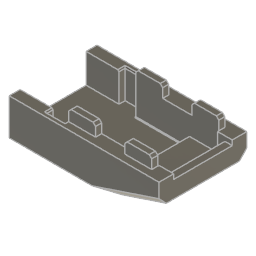
DiabolicParasite-Case-Top (Autodesk Fusion 360 design; units mm, degrees)
Autodesk Fusion 360 part; units mm, degrees
sketch "Skizze1" plane through (0, 0, 0) normal (0, 0, 1) x (1, 0, 0)
  line L0 (0, 0) -> (30.7, 0)
  line L1 (30.7, 0) -> (30.7, 18)
  line L2 (30.7, 18) -> (0, 18)
  line L3 (0, 18) -> (0, 0)
  dimension "d1" = 30.7
  dimension "d2" = 18
  constraint horizontal L0
  constraint vertical L1
  constraint horizontal L2
  constraint vertical L3
  constraint coincident L0.start L3.end
  measures "d1" distance of L0.start L0.end
  measures "d2" distance of L0.start L2.end
extrude "Extrusion1" add sketch "Skizze1" along normal blind 1.5
sketch "Skizze2" plane through (0, 0, 1.5) normal (0, 0, 1) x (-1, 0, 0)
  line L0 (0, -18) -> (0, 0)
  line L1 (0, 0) -> (-30.7, 0)
  line L2 (-30.7, 0) -> (-30.7, -18)
  line L3 (-30.7, -18) -> (0, -18)
  line L4 (-30.7, -18) -> (-10.7, -18)
  line L5 (-10.7, -18) -> (-10.7, -15)
  line L6 (-10.7, -15) -> (-30.7, -15)
  line L7 (-30.7, -15) -> (-30.7, -18)
  line L8 (-30.7, 0) -> (-10.7, 0)
  line L9 (-10.7, 0) -> (-10.7, -3)
  line L10 (-10.7, -3) -> (-30.7, -3)
  line L11 (-30.7, -3) -> (-30.7, 0)
  dimension "d5" = 20
  dimension "d6" = 3
  dimension "d7" = 20
  dimension "d8" = 3
  constraint horizontal L4
  constraint vertical L5
  constraint horizontal L6
  constraint vertical L7
  constraint coincident L2.end L3.start
  constraint horizontal L8
  constraint vertical L9
  constraint horizontal L10
  constraint vertical L11
  constraint coincident L1.end L2.start
  measures "d5" distance of L2.end L4.end
  measures "d6" distance of L2.end L6.end
  measures "d7" distance of L1.end L8.end
  measures "d8" distance of L1.end L10.end
extrude "Extrusion2" add sketch "Skizze2" along normal blind 6 contours L2 L3 L4 L5 L6 L7 | L1 L2 L8 L9 L10 L11
sketch "Skizze3" plane through (0, 0, 1.5) normal (0, 0, 1) x (-1, 0, 0)
  line L0 (-10.7, 0) -> (-10.7, -3)
  line L1 (-10.7, -3) -> (-30.7, -3)
  line L2 (-30.7, -3) -> (-30.7, -15)
  line L3 (-30.7, -15) -> (-10.7, -15)
  line L4 (-10.7, -15) -> (-10.7, -18)
  line L5 (-10.7, -18) -> (0, -18)
  line L6 (0, -18) -> (0, 0)
  line L7 (0, 0) -> (-10.7, 0)
  line L8 (-10.7, -18) -> (-10.7, -17)
  line L9 (-10.7, -17) -> (-7.5, -17)
  line L10 (-7.5, -17) -> (-7.5, -15.25)
  line L11 (-7.5, -15.25) -> (0, -15.25)
  line L12 (0, -15.25) -> (0, -18)
  line L13 (0, -18) -> (-10.7, -18)
  line L14 (-30.7, -9) -> (0.9, -9)
  line L15 (0, 0) -> (-10.7, 0)
  line L16 (0, -2.75) -> (0, 0)
  line L17 (-7.5, -2.75) -> (0, -2.75)
  line L18 (-7.5, -1) -> (-7.5, -2.75)
  line L19 (-10.7, -1) -> (-7.5, -1)
  line L20 (-10.7, 0) -> (-10.7, -1)
  dimension "d11" = 1
  dimension "d12" = 3.2
  dimension "d13" = 1.75
  constraint coincident L4.end L5.start
  constraint perpendicular L3 L8
  constraint perpendicular L4 L9
  constraint perpendicular L9 L10
  constraint coincident L6 L11.end
  constraint perpendicular L6 L11
  constraint coincident L5.end L6.start
  constraint midpoint L2 L14.start
  constraint perpendicular L6 L14
  constraint symmetric L4.end L14 L0.start
  constraint symmetric L8.end L14 L19.start
  constraint symmetric L9.end L14 L18.start
  constraint symmetric L10.end L14 L17.start
  constraint symmetric L11.end L14 L16.start
  constraint symmetric L5.end L14 L6.end
  measures "d11" distance of L4.end L8.end
  measures "d12" distance of L8.end L9.end
  measures "d13" distance of L9.end L10.end L6.end
extrude "Extrusion3" add sketch "Skizze3" along normal blind 6 contours L0 L6 L7 L15 L16 L17 L18 L19 L20 | L4 L5 L6 L8 L9 L10 L11 L12 L13
sketch "Skizze4" plane through (0, 0, 7.5) normal (0, 0, 1) x (-1, 0, 0)
  line L0 (-30.7, -15) -> (-30.7, -18)
  line L1 (-30.7, -18) -> (0, -18)
  line L2 (0, -18) -> (0, -15.25)
  line L3 (0, -15.25) -> (-7.5, -15.25)
  line L4 (-7.5, -15.25) -> (-7.5, -17)
  line L5 (-7.5, -17) -> (-10.7, -17)
  line L6 (-10.7, -17) -> (-10.7, -15)
  line L7 (-10.7, -15) -> (-30.7, -15)
sketch "Skizze5" plane through (0, 0, 7.5) normal (0, 0, 1) x (-1, 0, 0)
  line L0 (-10.7, -15) -> (-27.7, -15)
  line L1 (-27.7, -15) -> (-27.7, -16.5)
  line L2 (-27.7, -16.5) -> (-10.7, -16.5)
  line L3 (-10.7, -16.5) -> (-10.7, -15)
  line L4 (0, -18) -> (0, 0)
  line L5 (-27.7, -1.5) -> (-10.7, -1.5)
  line L6 (-10.7, -1.5) -> (-10.7, -3)
  line L7 (-10.7, -3) -> (-27.7, -3)
  line L8 (-27.7, -3) -> (-27.7, -1.5)
  point P0 (-30.7, -15)
  dimension "d18" = 17
  dimension "d19" = 1.5
  dimension "d20" = 3
  constraint horizontal L0
  constraint vertical L1
  constraint horizontal L2
  constraint vertical L3
  constraint coincident L4.end origin
  constraint perpendicular L0 L4
  measures "d18" distance of L0.start L0.end
  measures "d19" distance of L0.start L2.end
  measures "d20" distance of L0.end P0
extrude "Extrusion4" add sketch "Skizze5" along normal blind 2.4
chamfer "Fase1" distance 0.5 angle 45 4 edges at (10.7, 15.75, 9.9) (27.7, 15.75, 9.9) (10.7, 2.25, 9.9) (27.7, 2.25, 9.9)
extrude "Extrusion5" cut 1 faces at (2.5, 15.25, 5.5) along direction (0, 1, 0) blind 0.25
extrude "Extrusion6" cut 1 faces at (5, 2.75, 3.5) along direction (0, -1, 0) blind 0.25
sketch "Skizze6" plane through (0, 0, 1.5) normal (0, 0, 1) x (-1, 0, 0)
  line L0 (-7.5, -1) -> (-10.7, -1)
  line L1 (-10.7, -1) -> (-10.7, -3)
  line L2 (-10.7, -3) -> (-30.7, -3)
  line L3 (-30.7, -3) -> (-30.7, -15)
  line L4 (-30.7, -15) -> (-10.7, -15)
  line L5 (-10.7, -15) -> (-10.7, -17)
  line L6 (-10.7, -17) -> (-7.5, -17)
  line L7 (-7.5, -17) -> (-7.5, -15.5)
  line L8 (-7.5, -15.5) -> (0, -15.5)
  line L9 (0, -15.5) -> (0, -2.5)
  line L10 (0, -2.5) -> (-7.5, -2.5)
  line L11 (-7.5, -2.5) -> (-7.5, -1)
  line L12 (-30.7, -3) -> (-29.2, -3)
  line L13 (-29.2, -3) -> (-29.2, -15)
  line L14 (-29.2, -15) -> (-30.7, -15)
  line L15 (-30.7, -15) -> (-30.7, -3)
  dimension "d28" = 1.5
  constraint horizontal L12
  constraint vertical L13
  constraint horizontal L14
  constraint vertical L15
  constraint coincident L4 L13.end
  constraint coincident L2.end L3.start
  measures "d28" distance of L2.end L12.end
extrude "Extrusion7" add sketch "Skizze6" along normal blind 5 contours L2 L3 L4 L12 L13 L14 L15
extrude "Extrusion8" cut 1 faces at (7.5, 2, 5.5) along direction (-1, 0, 0) blind 0.5
extrude "Extrusion9" cut 1 faces at (7.5, 16.5, 3.5) along direction (-1, 0, 0) blind 0.5
extrude "Extrusion10" cut 1 faces at (4.6667, 15.5, 5.5) along direction (0, 1, 0) blind 0.25
extrude "Extrusion11" cut 1 faces at (4.6667, 2.5, 5.5) along direction (0, -1, 0) blind 0.25
sketch "Skizze7" plane through (0, 3, 0) normal (0, 1, 0) x (-1, 0, 0)
  line L0 (-30.7, 6.5) -> (-29.2, 6.5)
  line L1 (-29.2, 6.5) -> (-29.2, 1.5)
  line L2 (-29.2, 1.5) -> (-10.7, 1.5)
  line L3 (-10.7, 1.5) -> (-10.7, 9.4)
  line L4 (-10.7, 9.4) -> (-11.2, 9.9)
  line L5 (-11.2, 9.9) -> (-27.2, 9.9)
  line L6 (-27.2, 9.9) -> (-27.7, 9.4)
  line L7 (-27.7, 9.4) -> (-27.7, 7.5)
  line L8 (-27.7, 7.5) -> (-30.7, 7.5)
  line L9 (-30.7, 7.5) -> (-30.7, 6.5)
  line L10 (-27.7, 9.4) -> (-27.2, 9.9)
  line L11 (-27.2, 9.9) -> (-11.2, 9.9)
  line L12 (-11.2, 9.9) -> (-10.7, 9.4)
  line L13 (-10.7, 9.4) -> (-10.7, 1.5)
  line L14 (-27.7, 9.4) -> (-27.7, 1.5)
  line L15 (-27.7, 1.5) -> (-10.7, 1.5)
  constraint coincident L6.end L7.start
  constraint coincident L5.end L6.start
  constraint coincident L4.end L5.start
  constraint coincident L3.end L4.start
  constraint coincident L2.end L3.start
  constraint coincident L2 L14.end
  constraint perpendicular L2 L14
extrude "Extrusion12" cut sketch "Skizze7" against normal blind 0.25 contours L2 L3 L4 L5 L6 L7 L10 L11 L12 L13 L14 L15
sketch "Skizze8" plane through (0, 15, 0) normal (0, -1, 0) x (1, 0, 0)
  line L0 (29.2, 1.5) -> (29.2, 6.5)
  line L1 (29.2, 6.5) -> (30.7, 6.5)
  line L2 (30.7, 6.5) -> (30.7, 7.5)
  line L3 (30.7, 7.5) -> (27.7, 7.5)
  line L4 (27.7, 7.5) -> (27.7, 9.4)
  line L5 (27.7, 9.4) -> (27.2, 9.9)
  line L6 (27.2, 9.9) -> (11.2, 9.9)
  line L7 (11.2, 9.9) -> (10.7, 9.4)
  line L8 (10.7, 9.4) -> (10.7, 1.5)
  line L9 (10.7, 1.5) -> (29.2, 1.5)
  line L10 (27.7, 7.5) -> (27.7, 1.5)
  line L11 (27.7, 1.5) -> (10.7, 1.5)
  line L12 (10.7, 1.5) -> (10.7, 9.4)
  line L13 (10.7, 9.4) -> (11.2, 9.9)
  line L14 (11.2, 9.9) -> (27.2, 9.9)
  line L15 (27.2, 9.9) -> (27.7, 9.4)
  line L16 (27.7, 9.4) -> (27.7, 7.5)
extrude "Extrusion13" cut sketch "Skizze8" against normal blind 0.25 contours L4 L5 L6 L7 L8 L9 L10 L11 L12 L13 L14 L15 L16
extrude "Extrusion14" cut 1 faces at (7, 1.4167, 3.5) along direction (-1, 0, 0) blind 0.25
extrude "Extrusion15" cut 1 faces at (7, 16.5833, 3.5) along direction (-1, 0, 0) blind 0.25
chamfer "Fase3" distance 0.25 angle 45 4 edges at (8.725, 1, 7.5) (6.75, 1.625, 7.5) (6.75, 16.375, 7.5) (8.725, 17, 7.5)
sketch "Skizze9" plane through (0, 0, 9.9) normal (0, 0, 1) x (-1, 0, 0)
  line L0 (-27.2, -2.75) -> (-11.2, -2.75)
  line L1 (-11.2, -2.75) -> (-11.2, -1.5)
  line L2 (-11.2, -1.5) -> (-27.2, -1.5)
  line L3 (-27.2, -1.5) -> (-27.2, -2.75)
  line L4 (-22.2, -2.75) -> (-16.2, -2.75)
  line L5 (-16.2, -2.75) -> (-16.2, -1.5)
  line L6 (-16.2, -1.5) -> (-22.2, -1.5)
  line L7 (-22.2, -1.5) -> (-22.2, -2.75)
  line L8 (-22.2, -16.5) -> (-16.2, -16.5)
  line L9 (-16.2, -16.5) -> (-16.2, -15.25)
  line L10 (-16.2, -15.25) -> (-22.2, -15.25)
  line L11 (-22.2, -15.25) -> (-22.2, -16.5)
  point P0 (-27.7, -2.75)
  dimension "d49" = 6
  dimension "d50" = 5.5
  dimension "d51" = 1.25
  constraint horizontal L4
  constraint vertical L5
  constraint horizontal L6
  constraint vertical L7
  constraint coincident L2 L5.end
  constraint coincident L0 L4.start
  constraint horizontal L8
  constraint vertical L9
  constraint horizontal L10
  constraint vertical L11
  measures "d49" distance of L5 L7
  measures "d50" distance of L4.start P0
  measures "d51" distance of L8.start L10.end
extrude "Extrusion16" cut sketch "Skizze9" against normal blind 2.4 contours L0 L2 L4 L5 L6 L7 | L8 L9 L10 L11
chamfer "Fase4" distance 0.5 angle 45 4 edges at (22.2, 2.125, 9.9) (16.2, 2.125, 9.9) (16.2, 15.875, 9.9) (22.2, 15.875, 9.9)
sketch "Skizze10" plane through (0, 0, 1.5) normal (0, 0, 1) x (-1, 0, 0)
  line L0 (-29.2, -3) -> (-29.2, -15)
  line L1 (-29.2, -15) -> (-27.7, -15)
  line L2 (-27.7, -15) -> (-10.7, -15)
  line L3 (-10.7, -15) -> (-10.7, -15.25)
  line L4 (-10.7, -15.25) -> (-10.7, -17)
  line L5 (-10.7, -17) -> (-6.75, -17)
  line L6 (-6.75, -17) -> (-6.75, -15.75)
  line L7 (-6.75, -15.75) -> (0, -15.75)
  line L8 (0, -15.75) -> (0, -2.25)
  line L9 (0, -2.25) -> (-6.75, -2.25)
  line L10 (-6.75, -2.25) -> (-6.75, -1)
  line L11 (-6.75, -1) -> (-10.7, -1)
  line L12 (-10.7, -1) -> (-10.7, -2.75)
  line L13 (-10.7, -2.75) -> (-10.7, -3)
  line L14 (-10.7, -3) -> (-27.7, -3)
  line L15 (-27.7, -3) -> (-29.2, -3)
  line L16 (-29.2, -3) -> (-27.7, -3)
  line L17 (-27.7, -2.75) -> (-21.7, -2.75)
  line L18 (-29.2, -3) -> (-29.2, -15)
  line L19 (-29.2, -15) -> (-27.7, -15)
  line L20 (-27.7, -15) -> (-27.7, -15.25)
  line L21 (-27.7, -15.25) -> (-21.7, -15.25)
  line L22 (-21.7, -15.25) -> (-21.7, -2.75)
  line L23 (-27.7, -3) -> (-27.7, -2.75)
  dimension "d55" = 6
  dimension "d56" = 6
  constraint coincident L0.start L15.end
  constraint coincident L14.end L15.start
  constraint perpendicular L0 L17
  constraint coincident L0.end L1.start
  constraint coincident L1.end L2.start
  constraint perpendicular L1 L20
  constraint perpendicular L20 L21
  measures "d55" distance of L17.start L17.end
  measures "d56" distance of L20.end L21.end
extrude "Extrusion18" add sketch "Skizze10" along normal blind 2 contours L0 L1 L2 L14 L15 L16 L18 L19 L22 | L14 L17 L22 L23 | L2 L20 L21 L22
chamfer "Fase6" distance 3 distance2 9 1 edges at (30.7, 9, 0) measured on face at (30.7, 7, 2.1667)
chamfer "Fase7" distance 1.5 angle 45 2 edges at (26.2, 0, 1.5) (26.2, 18, 1.5)
sketch "Skizze11" plane through (0, 0, 0) normal (0, 0, -1) x (1, 0, 0)
  line L0 (16.9566, -18) -> (21.7, -16.5)
  line L1 (21.7, -16.5) -> (21.7, -1.5)
  line L2 (21.7, -1.5) -> (16.9566, 0)
  line L3 (16.9566, 0) -> (0, 0)
  line L4 (0, 0) -> (0, -18)
  line L5 (0, -18) -> (16.9566, -18)
  line L6 (1.2141, -8.8075) -> (4.2737, -10.5308)
  line L7 (4.2737, -10.5308) -> (4.2721, -9.2547)
  line L8 (4.2721, -9.2547) -> (13.5116, -9.2746)
  spline S0 degree 3 poles (13.5116, -9.2746) (13.4697, -9.4576) (13.3762, -9.6062) (13.3229, -9.7697) knots 0 0 0 0 1 1 1 1
  spline S1 degree 3 poles (13.3229, -9.7697) (13.022, -10.6918) (12.4198, -11.2426) (11.3356, -11.2485) knots 0 0 0 0 1 1 1 1
  line L9 (11.3356, -11.2485) -> (10.5675, -11.2692)
  spline S2 degree 3 poles (10.5675, -11.2692) (10.4017, -11.0954) (10.4168, -10.9819) (10.3217, -10.8317) knots 0 0 0 0 1 1 1 1
  spline S3 degree 3 poles (10.3217, -10.8317) (10.1903, -10.6244) (9.9419, -10.4277) (9.7381, -10.3457) knots 0 0 0 0 1 1 1 1
  spline S4 degree 3 poles (9.7381, -10.3457) (8.6591, -9.911) (7.5802, -10.5592) (7.5399, -11.7608) knots 0 0 0 0 1 1 1 1
  spline S5 degree 3 poles (7.5399, -11.7608) (7.6724, -13.4837) (9.8775, -13.9287) (10.5675, -12.1456) knots 0 0 0 0 1 1 1 1
  line L10 (10.5675, -12.1456) -> (11.6596, -12.1144)
  spline S6 degree 3 poles (11.6596, -12.1144) (12.302, -12.0867) (12.8976, -11.8491) (13.4441, -11.3899) knots 0 0 0 0 1 1 1 1
  spline S7 degree 3 poles (13.4441, -11.3899) (13.7999, -10.8974) (14.1556, -10.1496) (14.5114, -9.2735) knots 0 0 0 0 1 1 1 1
  line L11 (14.5114, -9.2735) -> (16.956, -9.2513)
  spline S8 degree 3 poles (16.956, -9.2513) (17.2824, -10.0163) (17.8277, -10.2894) (18.4423, -10.2766) knots 0 0 0 0 1 1 1 1
  spline S9 degree 3 poles (18.4423, -10.2766) (19.2203, -10.2605) (20.0125, -9.5959) (19.9455, -8.7505) knots 0 0 0 0 1 1 1 1
  spline S10 degree 3 poles (19.9455, -8.7505) (19.9306, -7.8243) (19.2679, -7.2245) (18.4499, -7.1909) knots 0 0 0 0 1 1 1 1
  spline S11 degree 3 poles (18.4499, -7.1909) (17.8244, -7.1652) (17.2457, -7.4602) (16.9343, -8.3207) knots 0 0 0 0 1 1 1 1
  line L12 (16.9343, -8.3207) -> (12.9518, -8.3145)
  spline S12 degree 3 poles (12.9518, -8.3145) (12.7451, -8.2038) (12.6152, -8.0651) (12.555, -7.9011) knots 0 0 0 0 1 1 1 1
  spline S13 degree 3 poles (12.555, -7.9011) (12.4826, -7.7094) (12.363, -7.5358) (12.2759, -7.3575) knots 0 0 0 0 1 1 1 1
  spline S14 degree 3 poles (12.2759, -7.3575) (11.6761, -6.1294) (10.5075, -5.4016) (9.0902, -5.3903) knots 0 0 0 0 1 1 1 1
  line L13 (9.0902, -5.3903) -> (8.5876, -5.3856)
  line L14 (8.5876, -5.3856) -> (8.5905, -4.5744)
  line L15 (8.5905, -4.5744) -> (5.9821, -4.5663)
  line L16 (5.9821, -4.5663) -> (5.9718, -7.1819)
  line L17 (5.9718, -7.1819) -> (8.6016, -7.1767)
  line L18 (8.6016, -7.1767) -> (8.595, -6.2677)
  spline S15 degree 3 poles (8.595, -6.2677) (10.3201, -6.3029) (11.3418, -7.0168) (11.7505, -8.3223) knots 0 0 0 0 1 1 1 1
  line L19 (11.7505, -8.3223) -> (4.2518, -8.3042)
  line L20 (4.2518, -8.3042) -> (4.2308, -7.0168)
  line L21 (4.2308, -7.0168) -> (1.2141, -8.8075)
extrude "Extrusion19" cut sketch "Skizze11" against normal blind 1 contours L6 L7 L8 S0 S1 L9 S2 S3 S4 S5 L10 S6 S7 L11 S8 S9 S10 S11 L12 S12 S13 S14 L13 L14 L15 L16 L17 L18 S15 L19 L20 L21
